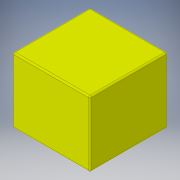
# Autodesk Inventor part: PowerCube
Saved by Autodesk Inventor 2016 (Build 200138000, 138)
## iProperties
Created: 2018-01-12
Part Number: PowerCube
Material: Generic
Document SubType Name: Modeling
Designer: New User
Density: 1 g/cm^3
Appearance: Default
Author: New User
Autodesk Inventor part; units mm, degrees
ref_plane "YZ Plane" through (0, 0, 0) normal (1, 0, 0) x (0, 1, 0)
ref_plane "XZ Plane" through (0, 0, 0) normal (0, 1, 0) x (-1, 0, 0)
ref_plane "XY Plane" through (0, 0, 0) normal (0, 0, 1) x (1, 0, 0)
sketch "Sketch1" plane through (0, 0, 0) normal (0, 1, 0) x (-1, 0, 0)
  line L0 (157.0743, 222.4264) -> (-173.1257, 222.4264)
  line L1 (-173.1257, 222.4264) -> (-173.1257, -107.7736)
  line L2 (-173.1257, -107.7736) -> (157.0743, -107.7736)
  line L3 (157.0743, -107.7736) -> (157.0743, 222.4264)
  point P0 (0, 0)
  dimension "d0" = 330.2
  constraints: 8 end point, 2 parallel, 2 perpendicular, 1 horizontal
  measures "d0" distance of L0.start L0.end
extrude "Extrusion1" add sketch "Sketch1" along normal blind 279.4
fillet "Fillet1" radius 6.35 12 edges at (8.0257, 279.4, 222.4264) (173.1257, 139.7, 222.4264) (173.1257, 279.4, 57.3264) (173.1257, 139.7, -107.7736) (173.1257, 0, 57.3264) (-157.0743, 139.7, 222.4264) (8.0257, 0, 222.4264) (-157.0743, 0, 57.3264) (8.0257, 0, -107.7736) (-157.0743, 139.7, -107.7736) (-157.0743, 279.4, 57.3264) (8.0257, 279.4, -107.7736)
body "Solid1"
